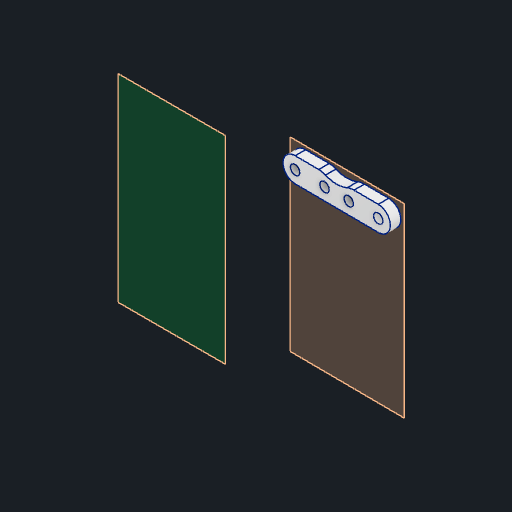
# Autodesk Inventor part: hip joint fix washer
Saved by Autodesk Inventor 2024.3 (Build 283343000, 343)
## iProperties
Created: 2022-06-18
Part Number: hip joint fix washer
Material: 알루미늄 6061
Document SubType Name: Sheet Metal
Designer: 박지훈
Density: 2.7 g/cm^3
Sheet Metal Rule: 기본값_mm
Appearance: 알루미늄 - 평지
Mass: 0.594108 g
Surface Area: 4.26854 cm^2
Volume: 0.22004 cm^3
Flat Pattern Width: 0.3 cm
Flat Pattern Length: 3.1 cm
Flat Pattern Area: 0.93 cm^2
Sheet Metal Width: 3.000 mm
Sheet Metal Length: 31.000 mm
Sheet Metal Area: 93.000 mm^2
Author: 박지훈
Autodesk Inventor part; units mm, degrees
ref_plane "YZ Plane" through (0, 0, 0) normal (1, 0, 0) x (0, 1, 0)
ref_plane "XZ Plane" through (0, 0, 0) normal (0, 1, 0) x (-1, 0, 0)
ref_plane "XY Plane" through (0, 0, 0) normal (0, 0, 1) x (1, 0, 0)
ref_plane "작업 평면1" through (23.0557, -14.7961, 15.1994) normal (0, 0, -1) x (-1, 0, 0)
ref_plane "작업 평면2" through (77.3136, -0.3645, 19.103) normal (-0.0064635, 0, 0.9999791) x (-0.9999791, 0, -0.0064635)
sketch "스케치3" plane through (77.3136, -0.3645, 19.103) normal (-0.0064635, 0, 0.9999791) x (-0.9999791, 0, -0.0064635)
  arc A0 (7.06, -22.04) -> (5.96, -20.94) centre (7.06, -20.94) ccw projected
  line L0 (7.06, -22.04) -> (7.06, -25) projected
  line L1 (7.06, -25) -> (15, -25) projected
  line L2 (15, -25) -> (15, -17.5339) projected
  arc A1 (15, -17.5339) -> (14.8713, -16.4701) centre (10.539, -17.5339) ccw projected
  line L3 (14.8713, -16.4701) -> (6.2746, 18.5407) projected
  arc A2 (6.2746, 18.5407) -> (-6.2746, 18.5407) centre (0, 17) ccw projected
  line L4 (-6.2746, 18.5407) -> (-14.8713, -16.4701) projected
  arc A3 (-14.8713, -16.4701) -> (-15, -17.5339) centre (-10.539, -17.5339) ccw projected
  line L5 (-15, -17.5339) -> (-15, -25) projected
  line L6 (-15, -25) -> (-7.06, -25) projected
  line L7 (-7.06, -25) -> (-7.06, -22.04) projected
  arc A4 (-5.96, -20.94) -> (-7.06, -22.04) centre (-7.06, -20.94) ccw projected
  line L8 (-5.96, -20.94) -> (5.96, -20.94) projected
  circle A5 centre (12, -23) radius 1.35 projected
  circle A6 centre (-12, -23) radius 1.35 projected
  line L9 (4.6428, 6.4789) -> (8.7217, -10.1327) projected
  arc A7 (5.516, -15.0285) -> (8.7217, -10.1327) centre (4.8371, -11.0865) ccw projected
  arc A8 (-5.516, -15.0285) -> (5.516, -15.0285) centre (0, 17) ccw projected
  arc A9 (-8.7217, -10.1327) -> (-5.516, -15.0285) centre (-4.8371, -11.0865) ccw projected
  line L10 (-8.7217, -10.1327) -> (-4.6428, 6.4789) projected
  arc A10 (-0.4945, 9.5163) -> (-4.6428, 6.4789) centre (-0.7582, 5.525) ccw projected
  arc A11 (-0.4945, 9.5163) -> (0.4945, 9.5163) centre (0, 17) ccw projected
  arc A12 (4.6428, 6.4789) -> (0.4945, 9.5163) centre (0.7582, 5.525) ccw projected
  circle A13 centre (0, 17) radius 4 projected
  circle A14 centre (3.5, -23) radius 1 projected
  circle A15 centre (-3.5, -23) radius 1 projected
  line L11 (7, -21) -> (7, -25) projected
  line L12 (-7, -21) -> (7, -21) projected
  line L13 (-7, -25) -> (-7, -21) projected
  line L14 (7, -25) -> (-7, -25) projected
  line L15 (12, -23) -> (-12, -23) construction
  line L16 (12, -19.5) -> (-12, -19.5)
  line L17 (-12, -26.5) -> (12, -26.5)
  arc A16 (12, -26.5) -> (12, -19.5) centre (12, -23) ccw
  arc A17 (-12, -19.5) -> (-12, -26.5) centre (-12, -23) ccw
  circle A18 centre (12, -23) radius 1.35
  circle A19 centre (3.5, -23) radius 1.35
  circle A20 centre (-3.5, -23) radius 1.35
  circle A21 centre (-12, -23) radius 1.35
  point P0 (77.4355, -0.3645)
  point P1 (0, -23)
  dimension "d12" = 7
  dimension "d13" = 2.7
  dimension "d14" = 2.7
  dimension "d15" = 2.7
  dimension "d16" = 2.7
  constraints: 8 end point, 6 centre point, 4 point on circle, 4 tangent, 1 coincident, 1 horizontal, 1 midpoint, 1 parallel
  measures "d12" diameter of A17
  measures "d13" diameter of A18
  measures "d14" diameter of A19
  measures "d15" diameter of A20
  measures "d16" diameter of A21
extrude "돌출3" add sketch "스케치3" along normal blind 3 contours L0 L1 A16 L17 A17 L6 L7 A4 L8 A0 | A0 L8 A4 L7 L6 A17 L5 L16 A16 L2 L1 L0 | L2 A16 | A17 L5 | L11 L14 L13 L12
sketch "스케치4" plane through (77.3136, -0.3645, 19.103) normal (0.0064635, 0, -0.9999791) x (-0.9999791, 0, -0.0064635)
  circle A0 centre (0.1001, 33.4603) radius 7.5 projected
  circle A1 centre (0.1001, 33.4603) radius 8
  point P0 (77.4355, 0.3645)
  dimension "d19" = 16
  constraints: 1 centre point, 1 coincident
  measures "d19" diameter of A1
extrude "돌출4" cut sketch "스케치4" against normal through all contours A0 | A1
fillet "모깎기2" radius 5 2 edges at (81.1477, 26.1355, 20.6278) (73.2599, 26.1355, 20.5768)
equation "\"TransitionRadius\" = BendRadius"
equation "\"BendRadius\" = 0.5"
